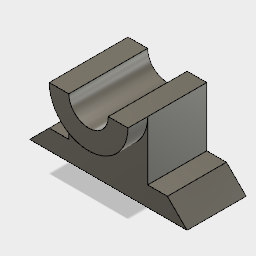
CAD Practice 1 (Autodesk Fusion 360 design; units mm, degrees)
Autodesk Fusion 360 part; units mm, degrees
sketch "Sketch1" plane through (0, 0, 0) normal (0, 0, 1) x (1, 0, 0)
  line L0 (0, 0) -> (80, 0)
  line L1 (80, 0) -> (70, 10)
  line L2 (70, 10) -> (60, 10)
  line L3 (60, 10) -> (60, 40)
  line L4 (0, 0) -> (10, 10)
  line L5 (10, 10) -> (20, 10)
  line L6 (20, 10) -> (20, 40)
  arc A0 (20, 40) -> (60, 40) centre (40, 40) ccw
  line L7 (20, 40) -> (30, 40)
  line L8 (30, 40) -> (20, 40)
  line L9 (50, 40) -> (60, 40)
  arc A1 (30, 40) -> (50, 40) centre (40, 40) ccw
  dimension "d1" = 80
  dimension "d2" = 10
  dimension "d3" = 45
  dimension "d4" = 10
  dimension "d5" = 45
  dimension "d6" = 40
  dimension "d8" = 30
  dimension "d9" = 30
  dimension "d10" = 10
  dimension "d11" = 20
  dimension "d15" = 10
  dimension "d16" = 20
  measures "d1" distance of L0.start L0.end
  measures "d2" distance of L0.start L4.end
  measures "d3" angle of L0 L4
  measures "d4" distance of L0.end L1.end
  measures "d5" angle of L0 L1
  measures "d6" distance of L3 L6
  measures "d8" distance of L2.end L3.end
  measures "d9" distance of L5.end L6.end
  measures "d10" distance of L4.end L5.end
  measures "d11" radius of A0
  measures "d15" distance of L6.end L7.end
  measures "d16" diameter of A1
extrude "Extrude1" add sketch "Sketch1" along normal blind 30 contours L0 L1 L2 L3 L4 L5 L6 A0
extrude "Extrude2" add sketch "Sketch1" along normal blind 40 contours A0 L7 L8 L9 A1
